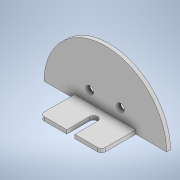
# Autodesk Inventor part: Rear
Saved by Autodesk Inventor 2021 (Build 250183000, 183)
## iProperties
Created: 2021-03-27
Part Number: Rear
Material: Generic
Document SubType Name: Modeling
Designer: cmzgt
Density: 1 g/cm^3
Appearance: Default
Author: cmzgt
Autodesk Inventor part; units mm, degrees
ref_plane "YZ Plane" through (0, 0, 0) normal (1, 0, 0) x (0, 1, 0)
ref_plane "XZ Plane" through (0, 0, 0) normal (0, 1, 0) x (-1, 0, 0)
ref_plane "XY Plane" through (0, 0, 0) normal (0, 0, 1) x (1, 0, 0)
sketch "Sketch1" plane through (0, 0, 0) normal (0, 0, 1) x (1, 0, 0)
  arc A0 (50.8, 0) -> (-50.8, 0) centre (0, 0) ccw
  line L0 (0, 0) -> (50.8, 0)
  line L1 (0, 0) -> (-50.8, 0)
  dimension "d0" = 101.6
  constraints: 4 end point, 2 horizontal, 2 point on circle, 1 centre point, 1 coincident
  measures "d0" diameter of A0
extrude "Extrusion1" add sketch "Sketch1" along normal blind 3.175
sketch "Sketch2" plane through (0, 0, 3.175) normal (0, 0, 1) x (1, 0, 0)
  arc A0 (50.8, 0) -> (-50.8, 0) centre (0, 0) ccw projected
  arc A1 (50.8, 0) -> (-50.8, 0) centre (0, 0) ccw projected
  line L0 (-50.8, 0) -> (50.8, 0) projected
  line L1 (0, 3.175) -> (0, 0) construction
  line L2 (0, 3.175) -> (25.4, 3.175)
  line L3 (25.4, 3.175) -> (25.4, 0)
  line L4 (-50.8, 0) -> (50.8, 0) projected
  line L5 (0, 3.175) -> (-25.4, 3.175)
  line L6 (-25.4, 3.175) -> (-25.4, 0)
  dimension "d6" = 25.4
  dimension "d7" = 3.175
  constraints: 10 end point, 2 symmetric about line, 1 horizontal, 1 perpendicular, 1 point on line, 1 vertical
  measures "d6" distance of L1.start L2.end
  measures "d7" distance between parallel lines of L0 L2
extrude "Extrusion2" add sketch "Sketch2" along normal blind 28.575 contours L0 L6 L5 L2 L3
fillet "Fillet1" radius 3.175 2 edges at (25.4, 1.5875, 31.75) (-25.4, 1.5875, 31.75)
sketch "Sketch3" plane through (-25.4, 3.175, 3.175) normal (0, 1, 0) x (1, 0, 0)
  line L0 (25.4, 3.175) -> (25.4, -28.575) construction
  line L1 (3.175, -28.575) -> (47.625, -28.575) construction
  line L2 (25.4, -28.575) -> (25.4, -6.35) construction
  line L3 (22.098, -25.273) -> (22.098, -9.652)
  line L4 (28.702, -9.652) -> (28.702, -25.273)
  arc A0 (22.098, -25.273) -> (28.702, -25.273) centre (25.4, -25.273) ccw
  arc A1 (28.702, -9.652) -> (22.098, -9.652) centre (25.4, -9.652) ccw
  line L5 (0, 0) -> (50.8, 0) projected
  line L6 (22.098, -25.273) -> (22.098, -28.575)
  line L7 (28.702, -25.273) -> (28.702, -28.575)
  line L8 (22.098, -28.575) -> (28.702, -28.575)
  point P0 (25.4, -17.4625)
  dimension "d11" = 6.35
  dimension "d12" = 6.604
  constraints: 16 end point, 6 point on circle, 6 point on line, 5 tangent, 2 centre point, 2 midpoint, 1 collinear, 1 parallel, 1 perpendicular
  measures "d11" distance from line of L5 L2.end
  measures "d12" distance between parallel lines of L4 L3
extrude "Extrusion3" cut sketch "Sketch3" against normal up to surface (3.175 mm away)
sketch "Sketch4" plane through (0, 0, 0) normal (0, 0, -1) x (-1, 0, 0)
  line L0 (0, 0) -> (0, 12.7) construction
  line L1 (0, 12.7) -> (12.7, 12.7) construction
  circle A0 centre (12.7, 12.7) radius 3.175
  circle A1 centre (-12.7, 12.7) radius 3.175
  dimension "d15" = 12.7
  dimension "d16" = 12.7
  dimension "d17" = 6.35
  constraints: 4 end point, 2 centre point, 1 coincident, 1 perpendicular, 1 symmetric about line, 1 vertical, 1 other
  measures "d15" distance of L0.start L0.end
  measures "d16" distance of L0.end L1.end
  measures "d17" diameter of A0
extrude "Extrusion4" cut sketch "Sketch4" against normal up to surface (3.175 mm away)
body "Solid1"
